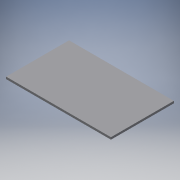
# Autodesk Inventor part: Pared Norte
Saved by Autodesk Inventor 2016 (Build 200138000, 138)
## iProperties
Created: 2015-11-12
Part Number: Pared Norte
Material: Generic
Document SubType Name: Modeling
Designer: serge
Density: 1 g/cm^3
Mass: 2.54e+06 g
Surface Area: 1.01524e+06 cm^2
Volume: 2.54e+06 cm^3
Appearance: Valor por defecto
Author: serge
Autodesk Inventor part; units mm, degrees
ref_plane "YZ Plane" through (0, 0, 0) normal (1, 0, 0) x (0, 1, 0)
ref_plane "XZ Plane" through (0, 0, 0) normal (0, 1, 0) x (-1, 0, 0)
ref_plane "XY Plane" through (0, 0, 0) normal (0, 0, 1) x (1, 0, 0)
sketch "Sketch1" plane through (0, 0, 0) normal (0, 0, 1) x (1, 0, 0)
  line L0 (-6993.5025, -3488.0368) -> (6.4975, -3488.0368)
  line L1 (6.4975, -3488.0368) -> (6.4975, 11.9632)
  line L2 (6.4975, 11.9632) -> (-6993.5025, 11.9632)
  line L3 (-6993.5025, 11.9632) -> (-6993.5025, -3488.0368)
  point P0 (0, 0)
  dimension "Largo" = 7000
  dimension "Alto" = 3500
  constraints: 8 end point, 2 parallel, 1 horizontal, 1 perpendicular
  measures "Largo" distance of L1.end L2.end
  measures "Alto" distance of L0.end L1.end
extrude "Extrusion1" add sketch "Sketch1" along normal blind 101.6
equation "\"Largo\" = PL_N"
equation "\"Alto\" = PA_N"
equation "\"Espesor\" = PE_N"
equation "\"PL_N\" = 7000"
equation "\"PA_N\" = 3500"
equation "\"PE_N\" = 101.6"
equation "\"PE_S\" = 101.6"
equation "\"PE_EO\" = 101.6"
equation "\"T_E\" = 101.6"
equation "\"lon_ve\" = 512.5"
equation "\"n_a\" = 3"
equation "\"t_a\" = 19.05"
equation "\"d_a\" = 128.125"
equation "\"lon_ho\" = 749"
equation "\"d_bor\" = 59.92"
equation "\"lon_gui\" = 187.25"
equation "\"esp_gui\" = 461.25"
equation "\"lon_ve2\" = 498.475"
equation "\"n_a2\" = 3"
equation "\"t_a2\" = 124.61875"
equation "\"d_a2\" = 124.61875"
equation "\"lon_ho2\" = 933.45"
equation "\"d_bor2\" = 74.676"
equation "\"lon_gui2\" = 233.3625"
equation "\"esp_gui2\" = 448.6275"
equation "\"UE_L\" = 2671"
equation "\"UE_A\" = 1025"
equation "\"UE_AN\" = 749"
equation "\"UC_L\" = 1314.45"
equation "\"UC_A\" = 996.95"
equation "\"UC_AN\" = 933.45"
equation "\"A_ET\" = 35"
equation "\"SEP_NS\" = 0"
equation "\"DSEG\" = 0"
equation "\"AEGEP_NS\" = 0"
equation "\"DNS\" = 749"
body "Solid1"
